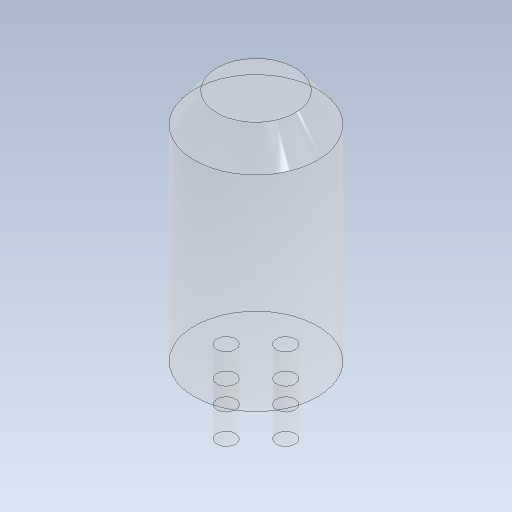
# Autodesk Inventor part: Flashbulb
Saved by Autodesk Inventor 2021 (Build 250183000, 183)
## iProperties
Created: 2021-08-11
Part Number: Flashbulb
Material: PET Plastic
Document SubType Name: Modeling
Designer: incep
Density: 1.541 g/cm^3
Appearance: Polycarbonate - Clear
Author: incep
Autodesk Inventor part; units mm, degrees
ref_plane "YZ Plane" through (0, 0, 0) normal (1, 0, 0) x (0, 1, 0)
ref_plane "XZ Plane" through (0, 0, 0) normal (0, 1, 0) x (-1, 0, 0)
ref_plane "XY Plane" through (0, 0, 0) normal (0, 0, 1) x (1, 0, 0)
sketch "Sketch1" plane through (0, 0, 0) normal (0, 0, 1) x (1, 0, 0)
  line L0 (-16.5, 55) -> (16.5, 55) construction
  line L1 (16.5, 55) -> (16.5, 0)
  line L2 (16.5, 0) -> (-16.5, 0)
  line L3 (-16.5, 0) -> (-16.5, 55)
  line L4 (-10.5, 63) -> (10.5, 63)
  line L5 (10.5, 63) -> (10.5, 55) construction
  line L6 (10.5, 55) -> (-10.5, 55) construction
  line L7 (-10.5, 55) -> (-10.5, 63) construction
  line L8 (-16.5, 55) -> (-10.5, 63)
  line L9 (10.5, 63) -> (16.5, 55)
  line L10 (0, 63) -> (0, 0)
  point P0 (0, 55)
  dimension "d0" = 33
  dimension "d1" = 55
  dimension "d2" = 21
  dimension "d3" = 63
  constraints: 22 end point, 4 parallel, 2 horizontal, 2 midpoint, 2 perpendicular, 1 collinear, 1 vertical, 1 vertical alignment
  measures "d0" distance of L1.end L2.end
  measures "d1" distance of L0.end L1.end
  measures "d2" distance of L4.start L4.end
  measures "d3" distance from line of L10.end L4
revolve "Revolution1" add sketch "Sketch1" angle 360 about axis through (0, 63, 0) along (0, -1, 0) contours L1 L2 L10 L4 L9
sketch "Sketch2" plane through (0, 0, 0) normal (0, -1, 0) x (1, 0, 0)
  circle A0 centre (0, -8) radius 2.5
  circle A1 centre (8, 0) radius 2.5
  circle A2 centre (0, 8) radius 2.5
  circle A3 centre (-8, 0) radius 2.5
  point P0 (0, 0)
  dimension "d5" = 5
  dimension "d6" = 8
  dimension "d9" = 360
  constraints: 4 centre point, 9 other
  measures "d5" diameter of A0
  measures "d6" distance of A0.centre point (0, 0)
extrude "Extrusion1" add sketch "Sketch2" along normal blind 14
body "Solid1"
